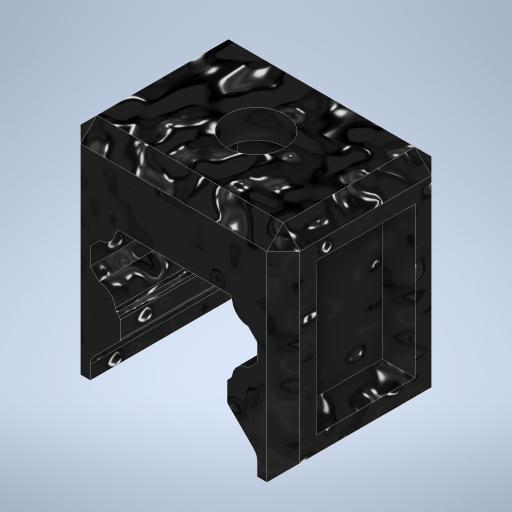
# Autodesk Inventor part: Tope Final
Saved by Autodesk Inventor 2023 (Build 270158000, 158)
## iProperties
Created: 2023-12-13
Part Number: Tope Final
Material: PET Plastic
Document SubType Name: Modeling
Designer: juanp
Density: 1.541 g/cm^3
Appearance: Black
Author: juanp
Autodesk Inventor part; units mm, degrees
ref_plane "YZ Plane" through (0, 0, 0) normal (1, 0, 0) x (0, 1, 0)
ref_plane "XZ Plane" through (0, 0, 0) normal (0, 1, 0) x (-1, 0, 0)
ref_plane "XY Plane" through (0, 0, 0) normal (0, 0, 1) x (1, 0, 0)
sketch "Sketch1" plane through (0, 0, 0) normal (0, 0, 1) x (1, 0, 0)
  arc A0 (-5.217, 1.3451) -> (-5.1032, 1.1142) centre (-4.8204, 1.397) ccw projected
  line L0 (-5.1032, 1.1142) -> (-4.8872, 0.8982) projected
  arc A1 (-4.77, 0.6153) -> (-4.8872, 0.8982) centre (-5.17, 0.6153) ccw projected
  line L1 (-4.77, 0.6153) -> (-4.77, -0.9467) projected
  arc A2 (-4.8872, -1.2296) -> (-4.77, -0.9467) centre (-5.17, -0.9467) ccw projected
  line L2 (-4.8872, -1.2296) -> (-7.2071, -3.5495) projected
  arc A3 (-7.2071, -3.5495) -> (-7.5, -4.2566) centre (-6.5, -4.2566) ccw projected
  line L3 (-7.5, -4.2566) -> (-7.5, -6.8) projected
  line L4 (-7.5, -6.8) -> (-6.8, -7.5) projected
  line L5 (-6.8, -7.5) -> (6.8, -7.5) projected
  line L6 (6.8, -7.5) -> (7.5, -6.8) projected
  line L7 (7.5, -6.8) -> (7.5, -4.2566) projected
  arc A4 (7.5, -4.2566) -> (7.2071, -3.5495) centre (6.5, -4.2566) ccw projected
  line L8 (7.2071, -3.5495) -> (4.8872, -1.2296) projected
  arc A5 (4.77, -0.9467) -> (4.8872, -1.2296) centre (5.17, -0.9467) ccw projected
  line L9 (4.77, -0.9467) -> (4.77, 0.6153) projected
  arc A6 (4.8872, 0.8982) -> (4.77, 0.6153) centre (5.17, 0.6153) ccw projected
  line L10 (4.8872, 0.8982) -> (5.1032, 1.1142) projected
  arc A7 (5.1032, 1.1142) -> (5.217, 1.3451) centre (4.8204, 1.397) ccw projected
  arc A8 (6.7419, 2.7529) -> (5.217, 1.3451) centre (6.8233, 1.1349) ccw projected
  line L11 (6.7419, 2.7529) -> (7.5, 3.511) projected
  line L12 (7.5, 3.511) -> (7.5, 5.049) projected
  line L13 (7.5, 5.049) -> (6.7304, 5.8186) projected
  arc A9 (5.2183, 7.2157) -> (6.7304, 5.8186) centre (6.8233, 7.436) ccw projected
  arc A10 (5.2183, 7.2157) -> (5.1049, 7.4441) centre (4.822, 7.1613) ccw projected
  line L14 (5.1049, 7.4441) -> (5.049, 7.5) projected
  line L15 (5.049, 7.5) -> (-5.049, 7.5) projected
  line L16 (-5.049, 7.5) -> (-5.1049, 7.4441) projected
  arc A11 (-5.1049, 7.4441) -> (-5.2183, 7.2157) centre (-4.822, 7.1613) ccw projected
  arc A12 (-6.7304, 5.8186) -> (-5.2183, 7.2157) centre (-6.8233, 7.436) ccw projected
  line L17 (-6.7304, 5.8186) -> (-7.5, 5.049) projected
  line L18 (-7.5, 5.049) -> (-7.5, 3.511) projected
  line L19 (-7.5, 3.511) -> (-6.7419, 2.7529) projected
  arc A13 (-5.217, 1.3451) -> (-6.7419, 2.7529) centre (-6.8233, 1.1349) ccw projected
  line L20 (-7.5, -5.5283) -> (-10, -5.5283)
  line L21 (-10, -5.5283) -> (-10, 14.2)
  line L22 (-10, 14.2) -> (10, 14.2)
  line L23 (10, 14.2) -> (10, -5.5283)
  line L24 (10, -5.5283) -> (7.5, -5.5283)
  arc A14 (-7.2778, -3.4788) -> (-7.6, -4.2566) centre (-6.5, -4.2566) ccw
  line L25 (-7.2778, -3.4788) -> (-4.9579, -1.1589)
  arc A15 (-4.9579, -1.1589) -> (-4.87, -0.9467) centre (-5.17, -0.9467) ccw
  line L26 (-4.87, -0.9467) -> (-4.87, 0.6153)
  arc A16 (-4.87, 0.6153) -> (-4.9579, 0.8275) centre (-5.17, 0.6153) ccw
  line L27 (-4.9579, 0.8275) -> (-5.1739, 1.0435)
  arc A17 (-5.3161, 1.3322) -> (-5.1739, 1.0435) centre (-4.8204, 1.397) ccw
  arc A18 (-5.3161, 1.3322) -> (-6.7848, 2.6544) centre (-6.8233, 1.1349) ccw
  line L28 (-6.7848, 2.6544) -> (-7.6, 3.4696)
  line L29 (-7.6, 3.4696) -> (-7.6, 5.0904)
  line L30 (-7.6, 5.0904) -> (-6.7736, 5.9168)
  arc A19 (-6.7736, 5.9168) -> (-5.3174, 7.2293) centre (-6.8233, 7.436) ccw
  arc A20 (-5.1756, 7.5148) -> (-5.3174, 7.2293) centre (-4.822, 7.1613) ccw
  line L31 (-5.1756, 7.5148) -> (-5.0904, 7.6)
  line L32 (-5.0904, 7.6) -> (5.0904, 7.6)
  line L33 (5.0904, 7.6) -> (5.1756, 7.5148)
  arc A21 (5.3174, 7.2293) -> (5.1756, 7.5148) centre (4.822, 7.1613) ccw
  arc A22 (5.3174, 7.2293) -> (6.7736, 5.9168) centre (6.8233, 7.436) ccw
  line L34 (6.7736, 5.9168) -> (7.6, 5.0904)
  line L35 (7.6, 5.0904) -> (7.6, 3.4696)
  line L36 (7.6, 3.4696) -> (6.7848, 2.6544)
  arc A23 (6.7848, 2.6544) -> (5.3161, 1.3322) centre (6.8233, 1.1349) ccw
  arc A24 (5.1739, 1.0435) -> (5.3161, 1.3322) centre (4.8204, 1.397) ccw
  line L37 (5.1739, 1.0435) -> (4.9579, 0.8275)
  arc A25 (4.9579, 0.8275) -> (4.87, 0.6153) centre (5.17, 0.6153) ccw
  line L38 (4.87, 0.6153) -> (4.87, -0.9467)
  arc A26 (4.87, -0.9467) -> (4.9579, -1.1589) centre (5.17, -0.9467) ccw
  line L39 (4.9579, -1.1589) -> (7.2778, -3.4788)
  arc A27 (7.6, -4.2566) -> (7.2778, -3.4788) centre (6.5, -4.2566) ccw
  line L40 (7.6, -4.2566) -> (7.6, -6.8414)
  line L41 (7.6, -6.8414) -> (6.8414, -7.6)
  line L42 (6.8414, -7.6) -> (-6.8414, -7.6)
  line L43 (-6.8414, -7.6) -> (-7.6, -6.8414)
  line L44 (-7.6, -6.8414) -> (-7.6, -4.2566)
  point P0 (0, 0)
  point P1 (-7.6, -5.5283)
  point P2 (7.6, -5.5283)
  dimension "d2" = 6.7
  dimension "d20" = 2.5
  dimension "d21" = 0.1
  constraints: 50 end point, 28 point on circle, 14 centre point, 2 midpoint, 2 perpendicular, 1 collinear, 1 horizontal, 1 parallel, 1 point on line, 33 other
  measures "d2" distance between parallel lines of L15 L22
  measures "d20" distance between parallel lines of L21 L3
  measures "d21" radial gap between concentric circles of A3 A14
extrude "Extrusion1" add sketch "Sketch1" against normal blind 15 contours L20 L21 L22 L23 L24 L40 A27 L39 A26 L38 A25 L37 A24 A23 L36 L35 L34 A22 A21 L33 L32 L31 A20 A19 L30 L29 L28 A18 A17 L27 A16 L26 A15 L25 A14 L44
chamfer "Chamfer1" distance 1.5 angle 45 10 edges at (-10, -5.5283, -7.5) (-10, 4.3358, -15) (-10, 4.3358, 0) (0, 14.2, -15) (0, 14.2, 0) (-10, 14.2, -7.5) (10, 4.3358, -15) (10, 4.3358, 0) (10, -5.5283, -7.5) (10, 14.2, -7.5)
sketch "Sketch3" plane through (-5.049, 7.6, 0) normal (0, -1, 0) x (1, 0, 0)
  line L0 (5.049, 0) -> (5.049, -15) construction
  circle A0 centre (5.049, -7.5) radius 2.65
  line L1 (10.1394, -15) -> (-0.0414, -15) projected
  dimension "d8" = 5.3
  constraints: 2 end point, 2 midpoint, 1 centre point, 1 vertical
  measures "d8" diameter of A0
extrude "Extrusion2" cut sketch "Sketch3" against normal blind 15
sketch "Sketch4" plane through (-5.049, 7.6, 0) normal (0, -1, 0) x (1, 0, 0)
  line L0 (1.049, -5.1906) -> (5.049, -2.8812)
  line L1 (5.049, -2.8812) -> (9.049, -5.1906)
  line L2 (9.049, -5.1906) -> (9.049, -9.8094)
  line L3 (9.049, -9.8094) -> (5.049, -12.1188)
  line L4 (5.049, -12.1188) -> (1.049, -9.8094)
  line L5 (1.049, -9.8094) -> (1.049, -5.1906)
  point P0 (5.049, 0)
  point P1 (5.049, -7.5)
  point P2 (5.049, -7.5)
  dimension "d11" = 8
  constraints: 12 end point, 1 coincident, 1 vertical, 13 other
  measures "d11" distance between parallel lines of L0 L3
extrude "Extrusion3" cut sketch "Sketch4" against normal blind 4
sketch "Sketch5" plane through (10, -4.0283, -13.5) normal (1, 0, 0) x (0, 0, -1)
  line L0 (0, 0) -> (-12, 0) projected
  line L1 (0, 16.7283) -> (0, 0) projected
  line L2 (-12, 16.7283) -> (0, 16.7283) projected
  line L3 (-12, 0) -> (-12, 16.7283) projected
  line L4 (-10.5, 15.2283) -> (-1.5, 15.2283)
  line L5 (-1.5, 15.2283) -> (-1.5, 1.5)
  line L6 (-1.5, 1.5) -> (-10.5, 1.5)
  line L7 (-10.5, 1.5) -> (-10.5, 15.2283)
  point P0 (-13.5, 4.0283)
  dimension "d14" = 1.5
  constraints: 8 end point, 3 other
  measures "d14" distance between parallel lines of L3 L7
extrude "Extrusion4" cut sketch "Sketch5" against normal blind 1.5 contours L4 L5 L6 L7
chamfer "Chamfer2" distance 1.5 angle 45 4 edges at (8.5, 4.3358, -3) (8.5, -2.5283, -7.5) (8.5, 11.2, -7.5) (8.5, 4.3358, -12)
mirror "Mirror1" about plane through (0, 0, 0) normal (1, 0, 0) of "Extrusion4", "Chamfer2"
body "Solid1"
